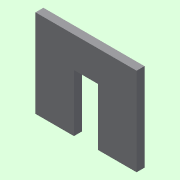
# Autodesk Inventor part: Distance_test_rig_insert
Saved by Autodesk Inventor 2015 (Build 190159000, 159)
## iProperties
Created: 2015-05-18
Part Number: Distance_test_rig_insert
Material: Generic
Document SubType Name: Modeling
Designer: Openlab
Density: 1 g/cm^3
Appearance: Default
Author: Openlab
Autodesk Inventor part; units mm, degrees
ref_plane "YZ Plane" through (0, 0, 0) normal (1, 0, 0) x (0, 1, 0)
ref_plane "XZ Plane" through (0, 0, 0) normal (0, 1, 0) x (-1, 0, 0)
ref_plane "XY Plane" through (0, 0, 0) normal (0, 0, 1) x (1, 0, 0)
sketch "Sketch1" plane through (0, 0, 0) normal (0, 1, 0) x (-1, 0, 0)
  line L0 (0.2295, -3) -> (23.2295, -3)
  line L1 (23.2295, -3) -> (23.2295, -23)
  line L2 (0.2295, -23) -> (0.2295, -3)
  line L3 (8.9795, -23) -> (8.9795, -10)
  line L4 (8.9795, -10) -> (14.4795, -10)
  line L5 (14.4795, -10) -> (14.4795, -23)
  line L6 (11.7295, -5) -> (11.7295, -18.3097) construction
  line L7 (23.2295, -23) -> (14.4795, -23)
  line L8 (8.9795, -23) -> (0.2295, -23)
  dimension "d4" = 23
  dimension "d5" = 20
  dimension "d8" = 5.5
  dimension "d9" = 13
  constraints: 18 end point, 3 parallel, 3 perpendicular, 2 vertical, 1 horizontal, 2 other
  measures "d4" distance of L1.end L2.start
  measures "d5" distance of L0.end L1.end
  measures "d8" distance of L3.end L4.end
  measures "d9" distance of L4.end L5.end
extrude "Extrusion1" add sketch "Sketch1" along normal blind 1.8
body "Solid1"
